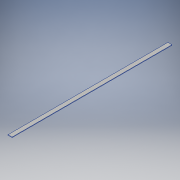
# Autodesk Inventor part: Solera de Al
Saved by Autodesk Inventor 2019 (Build 230136000, 136)
## iProperties
Created: 2019-11-05
Part Number: Solera de Al
Material: Aluminum 6061
Document SubType Name: Modeling
Designer: ErickBarcenas
Density: 2.7 g/cm^3
Appearance: Aluminum - Flat
Author: ErickBarcenas
Autodesk Inventor part; units mm, degrees
ref_plane "YZ Plane" through (0, 0, 0) normal (1, 0, 0) x (0, 1, 0)
ref_plane "XZ Plane" through (0, 0, 0) normal (0, 1, 0) x (-1, 0, 0)
ref_plane "XY Plane" through (0, 0, 0) normal (0, 0, 1) x (1, 0, 0)
sketch "Sketch1" plane through (0, 0, 0) normal (0, 1, 0) x (-1, 0, 0)
  line L0 (365.2982, 453.4736) -> (365.2982, -46.5264)
  line L1 (365.2982, 453.4736) -> (352.5982, 453.4736)
  line L2 (352.5982, 453.4736) -> (352.5982, -46.5264)
  line L3 (352.5982, -46.5264) -> (365.2982, -46.5264)
  point P0 (0, 0)
  dimension "d0" = 500
  dimension "d2" = 12.7
  constraints: 8 end point, 2 perpendicular, 1 horizontal, 1 vertical
  measures "d0" distance of L0.start L0.end
  measures "d2" distance of L0.start L1.end
extrude "Extrusion1" add sketch "Sketch1" along normal blind 1.6
body "Solid1"
